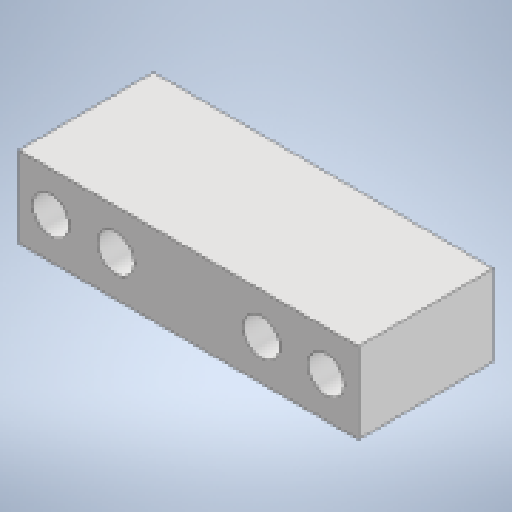
# Autodesk Inventor part: 부품78
Saved by Autodesk Inventor 2024 (Build 280153000, 153)
## iProperties
Created: 2024-09-09
Part Number: 부품78
Material: 일반
Document SubType Name: Modeling
Designer: Eungang
Mass: 5.09622 g
Surface Area: 45.7119 cm^2
Volume: 5.09622 cm^3
Density: 1 g/cm^3
Appearance: 기본값
Author: Eungang
Autodesk Inventor part; units mm, degrees
ref_plane "YZ Plane" through (0, 0, 0) normal (1, 0, 0) x (0, 1, 0)
ref_plane "XZ Plane" through (0, 0, 0) normal (0, 1, 0) x (-1, 0, 0)
ref_plane "XY Plane" through (0, 0, 0) normal (0, 0, 1) x (1, 0, 0)
sketch "스케치1" plane through (0, 0, 0) normal (0, 0, 1) x (1, 0, 0)
  circle A0 centre (-5.4019, -4.5) radius 1.35 projected
  circle A1 centre (5.4019, -4.5) radius 1.35 projected
  circle A2 centre (-10.2056, -4.5) radius 1.35 projected
  circle A3 centre (10.2056, -4.5) radius 1.35 projected
  line L0 (-3.0587, -2.4) -> (-3.0587, -6.5) projected
  arc A4 (-3.0587, -6.5) -> (-4.0587, -7.5) centre (-3.0587, -7.5) ccw projected
  line L1 (-4.0587, -7.5) -> (-12.6075, -7.5) projected
  line L2 (-12.6075, -7.5) -> (-12.6075, 7.5) projected
  line L3 (-12.6075, 7.5) -> (-17.6, 13.3735) projected
  line L4 (-17.6, 13.3735) -> (-17.6, 24.9) projected
  line L5 (-17.6, 24.9) -> (-12.2, 24.9) projected
  line L6 (-12.2, 24.9) -> (-12.2, 14.7038) projected
  arc A5 (-12.2, 14.7038) -> (-10.2, 12.7038) centre (-10.2, 14.7038) ccw projected
  line L7 (-10.2, 12.7038) -> (0, 12.7038) projected
  line L8 (0, 12.7038) -> (5.5223, 12.4914) projected
  line L9 (5.5223, 12.4914) -> (10.5959, 12.4914) projected
  arc A6 (10.5959, 12.4914) -> (12.5959, 14.4914) centre (10.5959, 14.4914) ccw projected
  line L10 (12.5959, 14.4914) -> (12.5959, 24.9) projected
  line L11 (12.5959, 24.9) -> (17.6, 24.9) projected
  line L12 (17.6, 24.9) -> (17.6, 13.3735) projected
  line L13 (17.6, 13.3735) -> (12.6075, 7.5) projected
  line L14 (12.6075, 7.5) -> (12.6075, -7.5) projected
  line L15 (12.6075, -7.5) -> (4.1413, -7.5) projected
  arc A7 (4.1413, -7.5) -> (3.1413, -6.5) centre (3.1413, -7.5) ccw projected
  line L16 (3.1413, -6.5) -> (3.1413, -2.4) projected
  arc A8 (3.1413, -2.4) -> (2.1413, -1.4) centre (3.1413, -1.4) ccw projected
  line L17 (2.1413, -1.4) -> (-2.0587, -1.4) projected
  arc A9 (-2.0587, -1.4) -> (-3.0587, -2.4) centre (-3.0587, -1.4) ccw projected
  circle A10 centre (-8.5, 10.1) radius 1.45 projected
  circle A11 centre (-15, 16.4) radius 1.45 projected
  circle A12 centre (15, 16.4) radius 1.45 projected
  circle A13 centre (8.5, 10.1) radius 1.45 projected
  line L18 (12.6075, -7.5) -> (-12.6075, -7.5)
  line L19 (-12.6075, -7.5) -> (-12.6075, -1.5)
  line L20 (-12.6075, -1.5) -> (12.6075, -1.5)
  line L21 (12.6075, -1.5) -> (12.6075, -7.5)
  line L22 (3.1413, -1.4) -> (3.0413, -1.4)
  line L23 (3.0413, -1.4) -> (3.0413, -1.5)
  line L24 (3.0413, -1.5) -> (3.1413, -1.5)
  line L25 (3.1413, -1.5) -> (3.1413, -1.4)
  line L26 (3.0413, -1.5) -> (-2.9587, -1.5)
  line L27 (-2.9587, -1.5) -> (-2.9587, -7.5)
  line L28 (-2.9587, -7.5) -> (3.0413, -7.5)
  line L29 (3.0413, -7.5) -> (3.0413, -1.5)
  point P0 (0, 0)
  point P1 (12.6075, -1.5)
  dimension "d0" = 6
  dimension "d1" = 0.1
  dimension "d2" = 0.1
  dimension "d3" = 6
  dimension "d4" = 6
  constraints: 24 end point, 6 parallel, 3 horizontal, 3 perpendicular, 1 point on line
  measures "d0" distance of L18.end L19.end
  measures "d1" distance of L24.end L23.end
  measures "d2" distance of L23.end L22.end
  measures "d3" distance of L28.end L27.end
  measures "d4" distance of L27.end L26.end
extrude "돌출1" add sketch "스케치1" along normal blind 30 contours A9 L20 L27 L18 A4 L0 | L0 A4 L1 L2 L20 A9 | L20 L29 L18 L27 | L20 A8 L16 A7 L18 L29 | L20 L14 L15 A7 L16 A8
sketch "스케치3" plane through (-12.6075, -7.5, 0) normal (0, -1, 0) x (1, 0, 0)
  line L0 (15.7488, 36) -> (15.7488, 30) projected
  line L1 (9.5488, 36) -> (9.5488, 30) projected
  line L2 (15.7488, 36) -> (15.6488, 36)
  line L3 (15.6488, 36) -> (15.6488, 35.9)
  line L4 (15.6488, 35.9) -> (15.7488, 35.9)
  line L5 (15.7488, 35.9) -> (15.7488, 36)
  line L6 (15.6488, 35.9) -> (9.6488, 35.9)
  line L7 (9.6488, 35.9) -> (9.6488, 29.9)
  line L8 (9.6488, 29.9) -> (15.6488, 29.9)
  line L9 (15.6488, 29.9) -> (15.6488, 35.9)
  line L10 (15.6488, 35.9) -> (9.6488, 35.9)
  line L11 (9.6488, 35.9) -> (9.6488, 36)
  line L12 (9.6488, 36) -> (15.6488, 36)
  line L13 (15.6488, 36) -> (15.6488, 35.9)
  line L14 (0, 30) -> (25.215, 30) projected
  line L15 (0, 0) -> (0, 30) projected
  line L16 (0, 15) -> (25.215, 15)
  line L17 (25.215, 0) -> (25.215, 30) projected
  line L18 (15.7488, -6) -> (15.7488, 0)
  line L19 (9.5488, -6) -> (9.5488, 0)
  line L20 (15.7488, -6) -> (15.6488, -6)
  line L21 (15.6488, -6) -> (15.6488, -5.9)
  line L22 (15.6488, -5.9) -> (15.7488, -5.9)
  line L23 (15.7488, -5.9) -> (15.7488, -6)
  line L24 (15.6488, -5.9) -> (9.6488, -5.9)
  line L25 (9.6488, -5.9) -> (9.6488, 0.1)
  line L26 (9.6488, 0.1) -> (15.6488, 0.1)
  line L27 (15.6488, 0.1) -> (15.6488, -5.9)
  line L28 (15.6488, -5.9) -> (9.6488, -5.9)
  line L29 (9.6488, -5.9) -> (9.6488, -6)
  line L30 (9.6488, -6) -> (15.6488, -6)
  line L31 (15.6488, -6) -> (15.6488, -5.9)
  line L32 (0, 0) -> (25.215, 0) projected
  point P0 (12.6075, 0)
  dimension "d11" = 0.1
  dimension "d12" = 0.1
  dimension "d13" = 6
  dimension "d14" = 6
  constraints: 54 end point, 13 symmetric about line, 6 parallel, 3 horizontal, 3 perpendicular, 2 midpoint
  measures "d11" distance of L4.end L3.end
  measures "d12" distance of L3.end L2.end
  measures "d13" distance of L8.end L7.end
  measures "d14" distance of L7.end L6.end
extrude "돌출2" add sketch "스케치3" against normal blind 6 contours L9 L14 L7 L6 | L9 L8 L7 L14 | L32 L25 L26 L27 | L27 L24 L25 L32 | L21 L30 L29 L24
sketch "스케치7" plane through (-12.6075, -7.5, 0) normal (0, -1, 0) x (1, 0, 0)
  line L0 (0, 30) -> (9.6488, 30) projected
  line L1 (0, 0) -> (0, 30) projected
  line L2 (0, 0) -> (9.6488, 0) projected
  line L3 (9.6488, 0) -> (9.6488, -6) projected
  line L4 (9.6488, -6) -> (15.6488, -6) projected
  line L5 (15.6488, -6) -> (15.6488, 0) projected
  line L6 (15.6488, 0) -> (25.215, 0) projected
  line L7 (25.215, 0) -> (25.215, 30) projected
  line L8 (15.6488, 30) -> (25.215, 30) projected
  line L9 (15.6488, 30) -> (15.6488, 35.9) projected
  line L10 (15.6488, 35.9) -> (9.6488, 35.9) projected
  line L11 (9.6488, 35.9) -> (9.6488, 30) projected
  line L12 (0, 0) -> (0, 30) projected
  line L13 (0, 0) -> (-2.3925, 0)
  line L14 (-2.3925, 0) -> (-2.3925, 30)
  line L15 (-2.3925, 30) -> (0, 30)
  line L16 (0, 30) -> (0, 0)
  line L17 (12.6075, 0) -> (12.6075, 30)
  line L18 (25.215, 0) -> (25.215, 30)
  line L19 (25.215, 0) -> (25.215, 30)
  line L20 (25.215, 0) -> (27.6075, 0)
  line L21 (27.6075, 0) -> (27.6075, 30)
  line L22 (27.6075, 30) -> (25.215, 30)
  line L23 (25.215, 30) -> (25.215, 0)
  dimension "d26" = 2.3925
  constraints: 22 end point, 4 symmetric about line, 2 parallel, 1 horizontal, 1 perpendicular, 1 vertical
  measures "d26" distance of L14.end L15.end
extrude "돌출6" add sketch "스케치7" against normal blind 6 contours L1 L13 L14 L15 | L22 L21 L20 L7
sketch "스케치8" plane through (-15, -7.5, 0) normal (-1, 0, 0) x (0, 0, 1)
  line L0 (0, 0) -> (30, 0) projected
  line L1 (15, 0) -> (15, 6)
  line L2 (30, 6) -> (0, 6) projected
  line L3 (15, 6) -> (12, 6)
  line L4 (12, 6) -> (12, 0)
  line L5 (12, 0) -> (15, 0)
  line L6 (15, 0) -> (15, 6)
  line L7 (15, 0) -> (18, 0)
  line L8 (18, 0) -> (18, 6)
  line L9 (18, 6) -> (15, 6)
  line L10 (15, 6) -> (15, 0)
  point P0 (0, 7.5)
  dimension "d29" = 3
  dimension "d30" = 3
  constraints: 18 end point, 4 parallel, 2 horizontal, 2 midpoint, 2 perpendicular, 2 point on line
  measures "d29" distance of L5.end L4.end
  measures "d30" distance of L9.end L8.end
extrude "돌출7" add sketch "스케치8" along normal blind 6
sketch "스케치9" plane through (-2.9587, -1.5, -6) normal (0, 1, 0) x (1, 0, 0)
  line L0 (6, -36) -> (17.9587, -36) projected
  line L1 (17.9587, -36) -> (17.9587, -6) projected
  line L2 (17.9587, -6) -> (6, -6) projected
  line L3 (6, -6) -> (6, 0) projected
  line L4 (6, 0) -> (0, 0) projected
  line L5 (0, 0) -> (0, -6) projected
  line L6 (0, -6) -> (-12.0413, -6) projected
  line L7 (-12.0413, -6) -> (-12.0413, -18) projected
  line L8 (-12.0413, -18) -> (-18.0413, -18) projected
  line L9 (-18.0413, -24) -> (-18.0413, -18) projected
  line L10 (-12.0413, -24) -> (-18.0413, -24) projected
  line L11 (-12.0413, -24) -> (-12.0413, -36) projected
  line L12 (0, -36) -> (-12.0413, -36) projected
  line L13 (0, -36) -> (0, -41.9) projected
  line L14 (0, -41.9) -> (6, -41.9) projected
  line L15 (6, -41.9) -> (6, -36) projected
  line L16 (2.9587, -6) -> (2.9587, -36)
  line L17 (17.9587, -18) -> (23.9587, -18)
  line L18 (23.9587, -24) -> (23.9587, -18)
  line L19 (17.9587, -24) -> (23.9587, -24)
  constraints: 8 end point, 4 symmetric about line, 1 vertical
extrude "돌출8" add sketch "스케치9" against normal blind 6 contours L1 L17 L18 L19
sketch "스케치10" plane through (15, -7.5, 0) normal (1, 0, 0) x (0, 0, -1)
  point P0 (0, 7.5)
sketch "스케치11" plane through (15, -7.5, 0) normal (1, 0, 0) x (0, 0, -1)
  circle A0 centre (-4.8357, 3) radius 1.35
  circle A1 centre (-9.6394, 3) radius 1.35
  circle A2 centre (-25.2469, 3) radius 1.35
  circle A3 centre (-20.4431, 3) radius 1.35
  point P0 (0, 7.5)
  constraints: 4 centre point, 8 other
extrude "돌출9" cut sketch "스케치11" against normal through all
